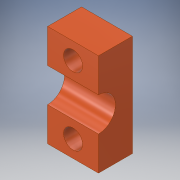
# Autodesk Inventor part: Hopper Smooth Rod Clamp
Saved by Autodesk Inventor 2018 (Build 220112000, 112)
## iProperties
Created: 2013-10-16
Part Number: Hopper Smooth Rod Clamp
Material: ABS Plastic
Document SubType Name: Modeling
Designer: Gabriel Smolnycki
Mass: 1.85281 g
Surface Area: 13.1911 cm^2
Volume: 1.74794 cm^3
Density: 1.06 g/cm^3
Appearance: Smooth - Light Orange
Sending System: SolidWorks 2017
Last Author: Gabriel Smolnycki
Last Saved: 2017-09-14
Author: Gabriel Smolnycki
Autodesk Inventor part; units mm, degrees
ref_plane "XZ Plane" through (0, 0, 0) normal (0, 1, 0) x (-1, 0, 0)
ref_plane "XY Plane" through (0, 0, 0) normal (0, 0, 1) x (1, 0, 0)
ref_plane "Work Plane1" through (-6, 0, 0) normal (1, 0, 0) x (0, 1, 0)
sketch "Sketch1" plane through (-6, 0, 0) normal (1, 0, 0) x (0, 1, 0)
  line L0 (-12, -8) -> (12, -8)
  arc A0 (-4, 0) -> (4, 0) centre (0, 0) ccw
  line L1 (-4, 0) -> (-12, 0)
  line L2 (12, -8) -> (12, 0)
  line L3 (-12, 0) -> (-12, -8)
  line L4 (12, 0) -> (4, 0)
  constraints: 10 end point, 3 equal length, 3 horizontal, 2 point on circle, 2 vertical, 1 centre point
extrude "Extrusion1" add sketch "Sketch1" along normal blind 12
hole "Hole2" at (0, -8, -8) direction (0, 0, 1) diameter 4.5 depth 8 tip angle 118
sketch "Sketch2" plane through (-6, -12, -8) normal (0, 0, -1) x (-1, 0, 0)
  point P0 (-6, 4)
hole "Hole1" at (0, 8, -8) direction (0, 0, 1) diameter 4.5 depth 8 tip angle 118
sketch "Sketch3" plane through (-6, -12, -8) normal (0, 0, -1) x (-1, 0, 0)
  point P0 (-6, 20)
body "Solid3"
